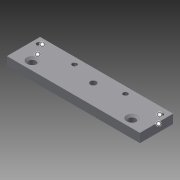
# Autodesk Inventor part: alu top plate
Saved by Autodesk Inventor 2015 SP1 (Build 190203100, 203)
## iProperties
Created: 2015-04-23
Part Number: alu top plate
Material: Generic
Document SubType Name: Modeling
Designer: ubik
Density: 1 g/cm^3
Appearance: Default
Author: ubik
Autodesk Inventor part; units mm, degrees
ref_plane "YZ Plane" through (0, 0, 0) normal (1, 0, 0) x (0, 1, 0)
ref_plane "XZ Plane" through (0, 0, 0) normal (0, 1, 0) x (-1, 0, 0)
ref_plane "XY Plane" through (0, 0, 0) normal (0, 0, 1) x (1, 0, 0)
sketch "Sketch1" plane through (0, 0, 0) normal (0, 0, 1) x (1, 0, 0)
  line L0 (0, 0) -> (120, 0)
  line L1 (120, 0) -> (120, 30)
  line L2 (120, 30) -> (0, 30)
  line L3 (0, 30) -> (0, 0)
  dimension "width" = 120
  dimension "d1" = 30
  constraints: 8 end point, 2 parallel, 1 horizontal, 1 perpendicular
  measures "width" distance of L1.end L2.end
  measures "d1" distance of L0.end L1.end
extrude "Extrusion1" add sketch "Sketch1" along normal blind 8
hole "Hole1" at (15, 8, 8) direction (0, 0, -1) diameter 6.5 end through all countersink diameter 10 countersink angle 90
hole "Hole2" at (105, 8, 8) direction (0, 0, -1) diameter 6.5 end through all countersink diameter 10 countersink angle 90
hole "Hole3" at (60, 18, 0) direction (0, 0, 1) diameter 16 depth 5
hole "Hole4" at (60, 18, 5) direction (0, 0, 1) diameter 5.5 end through all
hole "Hole5" at (5, 24, 8) direction (0, 0, -1) diameter 4.134 end through all thread size "M5x0.8" class "6H" standard "ANSI Metric M Profile"
hole "Hole6" at (115, 24, 8) direction (0, 0, -1) diameter 4.134 end through all thread size "M5x0.8" class "6H" standard "ANSI Metric M Profile"
pattern_linear "Rectangular Pattern1" count 2 spacing 32 along (1, 0, 0) of "Hole5"
pattern_linear "Rectangular Pattern2" count 2 spacing 32 along (-1, 0, 0) of "Hole6"
equation "\"d22\" = 0.5 * width"
body "Solid1"
